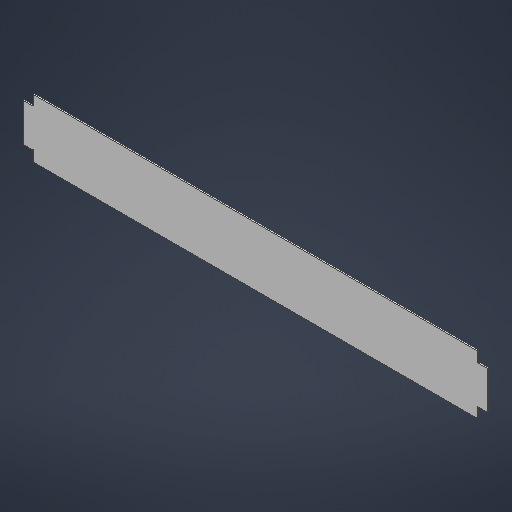
# Autodesk Inventor part: 内板
Saved by Autodesk Inventor 2025 (Build 290162000, 162)
## iProperties
Created: 2025-06-18
Part Number: 内板
Material: 常规
Document SubType Name: Modeling
Designer: XH
Density: 1 g/cm^3
Appearance: 默认
Author: XH
Autodesk Inventor part; units mm, degrees
ref_plane "YZ Plane" through (0, 0, 0) normal (1, 0, 0) x (0, 1, 0)
ref_plane "XZ Plane" through (0, 0, 0) normal (0, 1, 0) x (-1, 0, 0)
ref_plane "XY Plane" through (0, 0, 0) normal (0, 0, 1) x (1, 0, 0)
sketch "草图1" plane through (0, 0, 0) normal (0, 0, 1) x (1, 0, 0)
  line L0 (477.5, -60) -> (-477.5, -60)
  line L1 (-477.5, -60) -> (-477.5, 60)
  line L2 (-477.5, 60) -> (477.5, 60)
  line L3 (477.5, 60) -> (477.5, -60)
  line L4 (477.5, -60) -> (-477.5, 60) construction
  line L5 (-477.5, -60) -> (477.5, 60) construction
  line L6 (477.5, -40) -> (-477.5, -40) projected
  line L7 (477.5, 40) -> (-477.5, 40) projected
  line L8 (-457.5, 40) -> (-457.5, -40)
  line L9 (457.5, 40) -> (457.5, -40) projected
  line L10 (-455.5, -60) -> (-455.5, 60)
  line L11 (477.5, -39) -> (-477.5, -39)
  line L12 (477.5, 39) -> (-477.5, 39)
  line L13 (-475.5, 59.7487) -> (-475.5, -60)
  line L14 (475.5, 60) -> (475.5, -60)
  line L15 (455.5, 60) -> (455.5, -60)
  point P0 (0, 0)
  point P1 (457.5, -60)
  point P2 (457.5, 60)
  point P3 (-455.5, 40)
  point P4 (-455.5, -40)
  point P5 (457.5, 39)
  point P6 (-457.5, 39)
  point P7 (-457.5, -39)
  point P8 (457.5, -39)
  point P9 (-475.5, 39)
  point P10 (-475.5, -39)
  point P11 (475.5, -39)
  point P12 (475.5, 39)
  point P13 (-455.5, -39)
  point P14 (-455.5, 39)
  point P15 (455.5, -39)
  point P16 (455.5, 39)
  dimension "d0" = 120
  dimension "d1" = 955
  dimension "d4" = 1
  dimension "d5" = 1
  dimension "d6" = 2
  dimension "d7" = 2
  dimension "d8" = 2
  dimension "d9" = 2
  constraints: 26 end point, 11 point on line, 5 perpendicular, 4 parallel, 2 midpoint, 1 horizontal
  measures "d0" distance of L0.end L1.end
  measures "d1" distance of L1.end L2.end
  measures "d4" distance between parallel lines of L6 L11
  measures "d5" distance between parallel lines of L7 L12
  measures "d6" distance between parallel lines of L1 L13
  measures "d7" distance between parallel lines of L14 L3
  measures "d8" distance between parallel lines of L8 L10
  measures "d9" distance between parallel lines of L15 L9
extrude "拉伸1" add sketch "草图1" along normal blind 3 contours L0 L10 L6 L15 | L6 L10 L11 L15 | L11 L9 L12 L14 | L15 L12 L9 L11 | L11 L10 L12 L15 | L11 L8 L12 L10 | L12 L10 L7 L15 | L13 L12 L8 L11 | L7 L10 L2 L15
